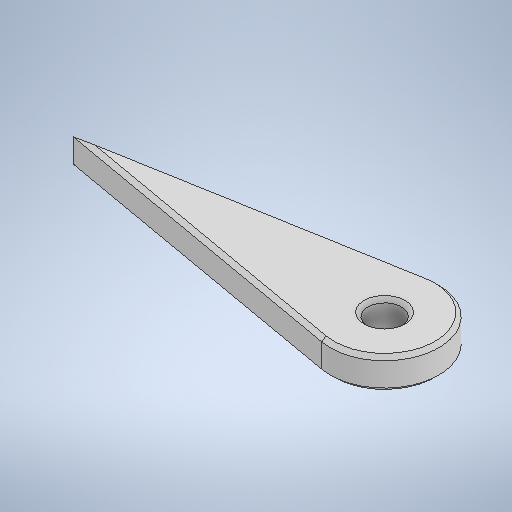
# Autodesk Inventor part: Pieza2
Saved by Autodesk Inventor 2025.1 (Build 291241000, 241)
## iProperties
Created: 2024-08-23
Part Number: Pieza2
Material: Genérico
Document SubType Name: Modeling
Designer: kraed
Density: 1 g/cm^3
Appearance: Valor por defecto
Author: kraed
Autodesk Inventor part; units mm, degrees
ref_plane "YZ Plane" through (0, 0, 0) normal (1, 0, 0) x (0, 1, 0)
ref_plane "XZ Plane" through (0, 0, 0) normal (0, 1, 0) x (-1, 0, 0)
ref_plane "XY Plane" through (0, 0, 0) normal (0, 0, 1) x (1, 0, 0)
sketch "Boceto1" plane through (0, 0, 0) normal (0, 1, 0) x (-1, 0, 0)
  circle A0 centre (0, 0) radius 2.7
  arc A1 (1.5138, 8.5673) -> (1.5138, -8.5673) centre (0, 0) ccw
  line L0 (1.5138, 8.5673) -> (50, 0)
  line L1 (50, 0) -> (1.5138, -8.5673)
  dimension "d0" = 5.4
  dimension "d1" = 6
  dimension "d2" = 50
  constraints: 4 end point, 2 centre point, 2 point on circle, 1 coincident, 1 concentric, 1 equal length, 1 horizontal alignment, 1 tangent
  measures "d0" diameter of A0
  measures "d1" radial gap between concentric circles of A1 A0
  measures "d2" distance of L0.end point (0, 0)
extrude "Extrusión1" add sketch "Boceto1" along normal blind 5
chamfer "Chaflán1" distance 0.6 angle 45 8 edges at (-25.7569, 5, 4.2836) (8.7, 5, 0) (-25.7569, 5, -4.2836) (-25.7569, 0, 4.2836) (8.7, 0, 0) (-25.7569, 0, -4.2836) (2.7, 5, 0) (2.7, 0, 0)
